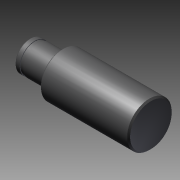
# Autodesk Inventor part: PSFRX15-30-F11-B3-P10
Saved by Autodesk Inventor 2016 (Build 200138000, 138)
## iProperties
Category: PARTsolutions
Company: MISUMI
Created: 2016-06-25
Part Number: PSFRX15-30-F11-B3-P10
Catalog Web Link: www.cadenas.de
Description: SFRX, PSFRX, SSFRX-Rotary Shafts - One End Stepped with Retaining Ring Groove -
Vendor: MISUMI
Document SubType Name: Modeling
Designer: psAdmin
Manufacturer: MISUMI
Mass: 49.146 g
Surface Area: 20.8313 cm^2
Volume: 6.14325 cm^3
Density: 8 g/cm^3
Material: ステンレス鋼
Appearance: 半つや出し
PSOL_IDENT_0: {$CADENAS_DATA\23d-libs\misumi\metric\11_rotary_shafts\sfrx.prj},282 {VTYP=3D},{NB=PSFRX15-30-F11-B3
PSOL_IDENT_1: -P10},{LINA=PSFRX15-30-F11-B3-P10},{NN=SFRX, PSFRX, SSFRX},{DATE=27.05.2016 14:10:13},{GEOMDATE=20.0
PSOL_IDENT_2: 1.2016 00:25:22},{VERSION=},{LINEID=70},{LINESUBID=-1},{WBVAR=MAT,ST,ALT1,L,F,B,P,ALT2,KC,A,WKC,C,K,
PSOL_IDENT_3: E,ALT3,FC,GALT3,WFC,J,W,V,ALT4,SFC,SG,AG,ALT5,UC}  {NB=PSFRX15-30-F11-B3-P10},{LINA=PSFRX15-30-F11-B
PSOL_IDENT_4: 3-P10},{KT=DUMMY},{PN=PSFRX15-30-F11-B3-P10},{TYPE=PSFRX},{MAT=S45C},{MATALG= 'S45C','S45C Equivalen
PSOL_IDENT_5: t', 'SUS304','SUS304' },{ST=ENP},{STALG= 'BO','Black Oxide', 'ENP','Electroless Nickel Plating' },{D=
PSOL_IDENT_6: 15},{ALT1=},{L=30.0},{LALG=[25:696/0.1]},{LMIN=25},{LMAX=696},{F=11.0},{FALG=[4:70/0.1]},{FMIN=4},{F
PSOL_IDENT_7: MAX=70},{B=3},{BMAX=9},{BMIN=2},{BALG=[2:9/1]},{P=10},{PALG=[5:10/1]},{PMAX=10},{PMAX1=10},{PMIN=5},
PSOL_IDENT_8: {PMIN1=3},{CIFC=0},{MM=1.15},{DD=9.6},{Y=800},{CC=0.5},{ALT2=},{ALT2ALG= '', 'w/o Key Grooves','KC','
PSOL_IDENT_9: with KC (Key Groove)','WKC','with WKC (Two Key Grooves)','KCWKC','with KC + WKC (Three Key Grooves)'
PSOL_IDENT_10: },{ALT2PN=},{KC=0.0},{KCALG=[0]},{KCMIN=0},{KCMAX1=25},{KCMAX2=15},{KCMAX3=10},{A=0.0},{AALG=[0]},{
PSOL_IDENT_11: AMIN=5},{AMAX1=30},{AMAX2=20},{AMAX3=15},{WKC=0.0},{WKCALG=[0]},{WKCMIN1=0},{WKCMIN2=0},{WKCMAX1=20}
PSOL_IDENT_12: ,{WKCMAX2=15},{C=0.0},{CALG=[0]},{CMIN=5},{CMAX1=25},{CMAX2=20},{K=0.0},{KALG=[0]},{KMIN1=0},{KMIN2=
PSOL_IDENT_13: 5},{KMAX1=25},{E=0.0},{EALG=[0]},{EMIN=5},{EMAX=30},{BB=5},{TT=3},{CIFR=0},{CIFKC=0},{CIFWKC=0},{CIF
PSOL_IDENT_14: K=0},{CIKC=0},{ALT3=},{ALT3ALG= '', 'w/o Set Screw Flat','FC','with FC (Adds a Set Screw Flat)','WFC'
PSOL_IDENT_15: ,'with WFC (Adds Two Set Screw Flats)','FCWFC','with FC + WFC (Adds Three Set Screw Flats)' },{ALT3P
PSOL_IDENT_16: N=},{FC=0},{FCALG=[0]},{FCMIN=0},{FCMAX=29},{GALT3=0},{GALT3ALG=[0]},{GALT3MIN=1},{GALT3MAX=30},{GAL
PSOL_IDENT_17: T3MAX2=24},{GALT3MAX3=27},{WFC=0},{WFCALG=[0]},{WFCMIN=0},{WFCMIN2=2},{WFCMAX=26},{WFCMAX2=-3},{WFCM
PSOL_IDENT_18: AX3=-4},{J=0},{JALG=[0]},{JMIN=1},{JMAX=27},{JMAX2=-2},{JMAX3=-5},{W=0},{WALG=[0]},{WMIN=0},{WMIN2=3
PSOL_IDENT_19: 2},{WMAX=27},{WMAX2=27},{V=0},{VALG=[0]},{VMIN=1},{VMAX=28},{VMAX2=28},{CIFCUT=0},{CIFFC=0},{ALT4=},
PSOL_IDENT_20: {ALT4ALG= '', 'w/o SFC (2 Set Screw Flats (Angle Specified))', 'SFC' , 'with SFC (2 Set Screw Flats
PSOL_IDENT_21: (Angle Specified))'},{ALT4PN=},{SFC=0},{SFCALG=[0]},{SFCMIN=0},{SFCMAX=29},{SG=0},{SGALG=[0]},{SGMIN=
PSOL_IDENT_22: 1},{SGMAX=30},{AG=0},{AGALG=[0]},{H=0},{CIFSFC=0},{ALT5=},{ALT5ALG= '','Not applicable' },{ALT5PN=},
PSOL_IDENT_23: {UC=0},{UCALG=[0]},{UCMIN=1},{UCMAX=24},{DDALT5=0},{LL1=0},{ERRORPN=},{ERRORALT2=OK},{ERRORALT23=OK}
PSOL_IDENT_24: ,{ERRORALT24=OK},{ERRORALT25=OK},{ERRORALT35=OK},{ERRORALT34=OK},{ERRORALT45=OK},{CIFKG=0},{KGMIN1=0
PSOL_IDENT_25: },{KGMAX1=0},{KGMIN2=0},{KGMAX2=0},{KGMIN3=0},{KGMAX3=0},{CIFKGC=0},{CIFKG1=1},{CIFKG2=0},{CIFKG3=0}
PSOL_IDENT_26: ,{CIFCALC1=0},{CIFCALC2=0},{CIFCALC3=0},{CIFKGPCUT=0},{PCUT3D=0}
NN: SFRX, PSFRX, SSFRX
NT: Rotary Shafts - One End Stepped with Retaining Ring Groove -
NB: PSFRX15-30-F11-B3-P10
NBSYN: $PN.
LINA: PSFRX15-30-F11-B3-P10
PN: PSFRX15-30-F11-B3-P10
MAT: S45C Equivalent
ST: Electroless Nickel Plating
D: 15
ALT1: w/o LKC (Changes L Tolerance)
L: 30.0
F: 11.0
B: 3
P: 10
Y: 800
ALT2: w/o Key Grooves
KC: 0.0
A: 0.0
WKC: 0.0
C: 0.0
K: 0.0
E: 0.0
ALT3: w/o Set Screw Flat
FC: 0
GALT3: 0
WFC: 0
J: 0
W: 0
V: 0
ALT4: w/o SFC (2 Set Screw Flats (Angle Specified))
SFC: 0
SG: 0
AG: 0
H: 0
ALT5: Not applicable
UC: 0
DDALT5: 0
LL1: 0
SUPPLIER: MISUMI
ARTICLENO: PSFRX15-30-F11-B3-P10
BOMINFO: PSFRX15-30-F11-B3-P10
CREATOR: CADENAS GmbH
Title: PSFRX15-30-F11-B3-P10
Author: Cadenas PARTsolutions
Comments: Rotary Shafts - One End Stepped with Retaining Ring Groove -
Autodesk Inventor part; units mm, degrees
ref_plane "YZ Plane" through (0, 0, 0) normal (1, 0, 0) x (0, 1, 0)
ref_plane "XZ Plane" through (0, 0, 0) normal (0, 1, 0) x (-1, 0, 0)
ref_plane "XY Plane" through (0, 0, 0) normal (0, 0, 1) x (1, 0, 0)
sketch "Sketch_1" plane through (0, 0, 0) normal (0, 0, 1) x (1, 0, 0)
  line L0 (30, 0) -> (-11, 0)
  line L1 (-11, 0) -> (-11, 4.5)
  line L2 (-11, 4.5) -> (-10.5, 5)
  line L3 (-10.5, 5) -> (-0.2, 5)
  arc A0 (-0.2, 5) -> (0, 5.2) centre (-0.2, 5.2) ccw
  line L4 (0, 5.2) -> (0, 7)
  line L5 (0, 7) -> (0.5, 7.5)
  line L6 (0.5, 7.5) -> (29.5, 7.5)
  line L7 (29.5, 7.5) -> (30, 7)
  line L8 (30, 7) -> (30, 0)
  line L9 (30, 0) -> (-11, 0)
  constraints: 20 end point, 2 point on circle, 1 centre point
revolve "Revolution1" add sketch "Sketch_1" angle 360 about axis through (30, 0, 0) along (1, 0, 0)
sketch "Sketch_40" plane through (0, 0, 0) normal (0, 0, 1) x (1, 0, 0)
  line L0 (1000, 0) -> (-1000, 0)
  line L1 (-9.15, 4.8) -> (-8, 4.8)
  line L2 (-8, 4.8) -> (-8, 20)
  line L3 (-8, 20) -> (-9.15, 20)
  line L4 (-9.15, 20) -> (-9.15, 4.8)
  constraints: 10 end point
revolve "Revolution2" cut sketch "Sketch_40" angle 360 about axis through (1000, 0, 0) along (1, 0, 0)
body "Solid1"
